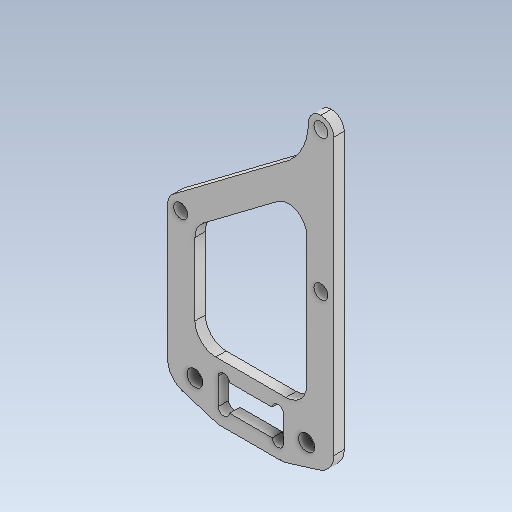
# Autodesk Inventor part: UpperArm_vertical_frame_01
Saved by Autodesk Inventor 2020.4 (Build 244396000, 396)
## iProperties
Created: 2021-09-07
Part Number: UpperArm_vertical_frame_01
Material: 一般
Document SubType Name: Modeling
Designer: aibay
Density: 1 g/cm^3
Appearance: 既定
Description: GFRP T2
Author: aibay
Autodesk Inventor part; units mm, degrees
ref_plane "YZ Plane" through (0, 0, 0) normal (1, 0, 0) x (0, 1, 0)
ref_plane "XZ Plane" through (0, 0, 0) normal (0, 1, 0) x (-1, 0, 0)
ref_plane "XY Plane" through (0, 0, 0) normal (0, 0, 1) x (1, 0, 0)
sketch "スケッチ2" plane through (0, 0, 0) normal (0, 0, 1) x (1, 0, 0)
  circle A0 centre (0, 0) radius 1.35
  line L0 (2.5, 0) -> (2.5, -56)
  circle A1 centre (0, 0) radius 2.4
  arc A2 (2.5, 0) -> (0, 2.4) centre (-0.046276, -0.150287) ccw
  arc A3 (0, 2.4) -> (-2.4, 0) centre (0, 0) ccw
  circle A4 centre (0, -27) radius 1.35
  circle A5 centre (-27, -27) radius 1.35
  line L1 (-7.25, -59) -> (2.5, -56)
  line L2 (-19.75, -56) -> (-19.75, -59)
  line L3 (-19.75, -59) -> (-29.5, -56)
  line L4 (-19.75, -59) -> (-7.25, -59)
  line L5 (-29.5, -56) -> (-29.5, -27)
  circle A6 centre (-8.3, -56) radius 1.05
  circle A7 centre (-8.3, -51) radius 1.05
  circle A8 centre (-18.7, -51) radius 1.05
  circle A9 centre (-18.7, -56) radius 1.05
  circle A10 centre (-2.75, -53.5) radius 1.55
  circle A11 centre (-24.25, -53.5) radius 1.55
  line L6 (-6.75, -48) -> (-20.25, -48)
  line L7 (-29.5, -27) -> (-27, -27)
  line L8 (-27, -27) -> (-28.554237, -25.041851)
  circle A12 centre (-27, -27) radius 2.5
  line L9 (-24.25, -44) -> (-24.25, -30.090988)
  line L10 (-2.75, -44) -> (-2.75, -18.930071)
  line L11 (-8.354493, -16.133446) -> (-22.655135, -26.894845)
  arc A13 (-28.554237, -25.041851) -> (-29.5, -27) centre (-27, -27) ccw
  line L12 (-28.554237, -25.041851) -> (-6.048598, -8.106096)
  arc A14 (-6.048598, -8.106096) -> (-2.4, 0) centre (-13.536142, 0.138263) ccw
  line L13 (-7.25, -56) -> (-7.25, -59)
  line L14 (-19.75, -56) -> (-7.25, -56)
  line L15 (-7.25, -56) -> (-7.25, -51)
  line L16 (-7.25, -51) -> (-19.75, -51)
  line L17 (-19.75, -51) -> (-19.75, -56)
  line L18 (-19.8, -50.95) -> (-7.2, -50.95)
  line L19 (-7.2, -50.95) -> (-7.2, -56.05)
  line L20 (-7.2, -56.05) -> (-19.8, -56.05)
  line L21 (-19.8, -56.05) -> (-19.8, -50.95)
  circle A15 centre (-18.7, -51) radius 1.1
  circle A16 centre (-8.3, -51) radius 1.1
  circle A17 centre (-18.7, -56) radius 1.1
  circle A18 centre (-8.3, -56) radius 1.1
  line L22 (2.5, -56) -> (-29.5, -56)
  circle A19 centre (-16, 1) radius 10.5
  arc A20 (-22.655135, -26.894845) -> (-24.25, -30.090988) centre (-20.25, -30.090988) ccw
  arc A21 (-24.25, -44) -> (-20.25, -48) centre (-20.25, -44) ccw
  arc A22 (-6.75, -48) -> (-2.75, -44) centre (-6.75, -44) ccw
  arc A23 (-2.75, -18.930071) -> (-8.354493, -16.133446) centre (-6.25, -18.930071) ccw
  point P0 (-2.75, -48)
  point P1 (-24.25, -48)
  point P2 (-24.25, -28.095)
  point P3 (-2.75, -11.916)
  point P4 (-19.798863, -50.95)
  point P5 (-17.601137, -50.95)
  point P6 (-9.398863, -50.95)
  point P7 (-7.201137, -50.95)
  point P8 (-7.201137, -56.05)
  point P9 (-9.398863, -56.05)
  point P10 (-17.601137, -56.05)
  point P11 (-19.798863, -56.05)
  dimension "d0" = 2.7
  dimension "d1" = 56
  dimension "d2" = 32
  dimension "d3" = 4.8
  dimension "d6" = 2.7
  dimension "d7" = 2.7
  dimension "d10" = 29
  dimension "d11" = 5
  dimension "d13" = 3.1
  dimension "d14" = 2.5
  dimension "d15" = 51.56
  dimension "d18" = 28.166
  dimension "d23" = 0.05
  dimension "d25" = 0.05
  dimension "d27" = 0.05
  dimension "d29" = 0.05
  dimension "d34" = 21
  dimension "d35" = 4
  dimension "d36" = 3.5
  constraints: 46 end point, 20 centre point, 18 point on circle, 11 vertical, 10 horizontal, 10 tangent, 8 point on line, 5 parallel, 3 coincident, 3 horizontal alignment, 3 perpendicular, 2 equal radius, 1 concentric, 25 other
  measures "d0" diameter of A0
  measures "d1" distance of L0.start L0.end
  measures "d2" distance of L0.end L3.end
  measures "d3" diameter of A1
  measures "d6" diameter of A4
  measures "d7" diameter of A5
  measures "d10" distance of L3.end L5.end
  measures "d11" distance of L15.end L13.start
  measures "d13" diameter of A11
  measures "d14" distance of L7.end L8.end
  measures "d15" angle of L8 L7
  measures "d18" distance of L8.end L12.end
  measures "d23" radial gap between concentric circles of A8 A15
  measures "d34" diameter of A19
  measures "d35" radius of A20
  measures "d36" radius of A23
sketch "スケッチ2 outline for 押し出し2" plane through (0, 0, 0) normal (0, 0, 1) x (1, 0, 0)
  line L0 (-29.5, -27) -> (-29.5, -56)
  arc A0 (-28.554237, -25.041851) -> (-29.5, -27) centre (-27, -27) ccw
  line L1 (-29.5, -56) -> (-19.75, -59)
  line L2 (-6.048598, -8.106096) -> (-28.554237, -25.041851)
  line L3 (-19.75, -59) -> (-7.25, -59)
  arc A1 (-2.4, 0) -> (-6.048598, -8.106096) centre (-13.536142, 0.138263) cw
  line L4 (-7.25, -59) -> (2.5, -56)
  arc A2 (0, 2.4) -> (-2.4, 0) centre (0, 0) ccw
  line L5 (2.5, -56) -> (2.5, 0)
  arc A3 (2.5, 0) -> (0, 2.4) centre (-0.046276, -0.150287) ccw
  circle A4 centre (-24.25, -53.5) radius 1.55
  line L6 (-6.75, -48) -> (-20.25, -48)
  arc A5 (-2.75, -44) -> (-6.75, -48) centre (-6.75, -44) cw
  line L7 (-2.75, -18.930071) -> (-2.75, -44)
  arc A6 (-8.354493, -16.133446) -> (-2.75, -18.930071) centre (-6.25, -18.930071) cw
  line L8 (-22.655135, -26.894845) -> (-8.354493, -16.133446)
  arc A7 (-24.25, -30.090988) -> (-22.655135, -26.894845) centre (-20.25, -30.090988) cw
  line L9 (-24.25, -44) -> (-24.25, -30.090988)
  arc A8 (-20.25, -48) -> (-24.25, -44) centre (-20.25, -44) cw
  line L10 (-19.798863, -56.05) -> (-19.8, -50.95)
  arc A9 (-17.601137, -56.05) -> (-19.798863, -56.05) centre (-18.7, -56) cw
  line L11 (-9.398863, -56.05) -> (-17.601137, -56.05)
  arc A10 (-7.2, -56.05) -> (-9.398863, -56.05) centre (-8.299432, -55.999405) cw
  line L12 (-7.201137, -50.95) -> (-7.2, -56.05)
  arc A11 (-9.398863, -50.95) -> (-7.201137, -50.95) centre (-8.3, -51) cw
  line L13 (-17.601137, -50.95) -> (-9.398863, -50.95)
  arc A12 (-19.8, -50.95) -> (-17.601137, -50.95) centre (-18.700568, -51.000595) cw
  circle A13 centre (-2.75, -53.5) radius 1.55
  circle A14 centre (-27, -27) radius 1.35
  circle A15 centre (0, -27) radius 1.35
  circle A16 centre (0, 0) radius 1.35
extrude "押し出し2" add sketch "スケッチ2 outline for 押し出し2" along normal blind 2
fillet "フィレット3" radius 4 4 edges at (-29.5, -56, 1) (-19.75, -59, 1) (-7.25, -59, 1) (2.5, -56, 1)
